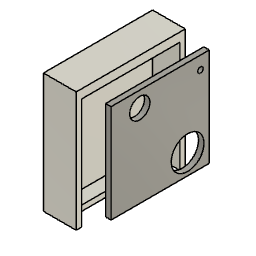
Configuration 1 (Autodesk Fusion 360 design; units mm, degrees)
Autodesk Fusion 360 part; units mm, degrees
note: some values were not read from the file. Set by a fixed rule: which sketch regions a step uses.
sketch "Sketch1" plane through (0, 0, 0) normal (1, 0, 0) x (0, 1, 0)
  line L0 (0, 0) -> (40, 0)
  line L1 (0, 0) -> (0, 43.9262)
  line L2 (0, 43.9262) -> (40, 43.9262)
  line L3 (40, 43.9262) -> (40, 0)
  dimension "d1" = 40
  constraint coincident L0.start L1.start
  constraint horizontal L0
  constraint perpendicular L0 L1
  constraint perpendicular L1 L2
  constraint perpendicular L0 L3
  measures "d1" distance of L0.start L0.end
extrude "Extrude1" add sketch "Sketch1" along normal blind 2 makes body 1
sketch "Sketch2" plane through (2, 0, 0) normal (1, 0, 0) x (0, 1, 0)
  line L0 (0, 0) -> (40, 0)
  line L1 (40, 0) -> (40, 43.9262)
  line L2 (40, 43.9262) -> (0, 43.9262)
  line L3 (0, 43.9262) -> (0, 0)
  line L4 (0, 43.9262) -> (40, 43.9262)
  line L5 (40, 0) -> (38, 0)
  line L6 (38, 40.6923) -> (2, 40.6923)
  line L7 (2, 40.6923) -> (2, 0)
  line L8 (0, 0) -> (2, 0)
  line L9 (38, 40.6923) -> (38, 0)
  constraint coincident L2.end L3.start
  constraint coincident L1.end L2.start
  constraint coincident L0.end L1.start
  constraint coincident L0 L5.end
  constraint perpendicular L1 L5
  constraint perpendicular L1 L6
  constraint coincident L0 L7.end
  constraint perpendicular L0 L7
  constraint coincident L0.start L3.end
  constraint perpendicular L5 L9
extrude "Extrude2" add sketch "Sketch2" along normal blind 10 contours L0 L1 L2 L3 L4 L5 L6 L7 L8 L9 bodies 1
sketch "Sketch3" plane through (2, 0, 0) normal (1, 0, 0) x (0, 1, 0)
  line L0 (38, 0) -> (38, 40.6923)
  line L1 (38, 40.6923) -> (2, 40.6923)
  line L2 (2, 40.6923) -> (2, 0)
  line L3 (2, 0) -> (38, 0)
  line L4 (2, 0) -> (38, 0)
  line L5 (38, 2) -> (2, 2)
  line L6 (2, 0) -> (2, 2)
  line L7 (38, 0) -> (38, 2)
  constraint coincident L2.end L3.start
  constraint coincident L0.start L3.end
  constraint coincident L2 L5.end
  constraint perpendicular L2 L5
  constraint perpendicular L5 L7
extrude "Extrude3" add sketch "Sketch3" along normal blind 5 contours L0 L2 L3 L4 L5 L6 L7 bodies 1
sketch "Sketch4" plane through (2, 0, 0) normal (1, 0, 0) x (0, 1, 0)
  line L0 (2, 2) -> (38, 2)
  line L1 (38, 2) -> (38, 40.6923)
  line L2 (38, 40.6923) -> (2, 40.6923)
  line L3 (2, 40.6923) -> (2, 2)
  line L4 (50, 0) -> (86, 0)
  line L5 (86, 0) -> (86, 36)
  line L6 (86, 36) -> (50, 36)
  line L7 (50, 36) -> (50, 0)
  dimension "d8" = 36
  dimension "d9" = 36
  constraint perpendicular L1 L4
  constraint perpendicular L4 L5
  constraint perpendicular L5 L6
  constraint perpendicular L4 L7
  measures "d8" distance of L4.start L4.end
  measures "d9" distance of L4.end L5.end
extrude "Extrude4" add sketch "Sketch4" along normal blind 2 separate body contours L4 L5 L6 L7 makes body 2
sketch "Sketch5" plane through (4, 0, 0) normal (1, 0, 0) x (0, 1, 0)
  line L0 (50, 36) -> (50, 0)
  line L1 (50, 0) -> (86, 0)
  line L2 (86, 0) -> (86, 36)
  line L3 (86, 36) -> (50, 36)
  circle A0 centre (78.0575, 7.3809) radius 6
  circle A1 centre (82.7779, 31.2818) radius 1
  dimension "d12" = 12
  dimension "d13" = 2
  measures "d12" diameter of A0
  measures "d13" diameter of A1
extrude "Extrude5" cut sketch "Sketch5" against normal blind 2 contours A0 | A1 bodies 2
move_body "Move1" bodies 2 to x (1, 0, 0) y (0, 1, 0) z (0, 0, 1) at (15, -48, 2)
move_body "Move2" bodies 2 to x (1, 0, 0) y (0, 1, 0) z (0, 0, 1) at (-6, 0, 0)
sketch "Sketch6" plane through (13, 0, 0) normal (1, 0, 0) x (0, 1, 0)
  circle A0 centre (30.0575, 9.3809) radius 6
  circle A1 centre (34.7779, 33.2818) radius 1
  line L0 (2, 38) -> (2, 2)
  line L1 (2, 2) -> (38, 2)
  line L2 (38, 2) -> (38, 38)
  line L3 (38, 38) -> (2, 38)
move_body "Move3" bodies 2 to x (1, 0, 0) y (0, 1, 0) z (0, 0, 1) at (18, 0, 0)
sketch "Sketch7" plane through (31, 0, 0) normal (1, 0, 0) x (0, 1, 0)
  circle A0 centre (30.0575, 9.3809) radius 6
  circle A1 centre (34.7779, 33.2818) radius 1
  line L0 (2, 38) -> (2, 2)
  line L1 (2, 2) -> (38, 2)
  line L2 (38, 2) -> (38, 38)
  line L3 (38, 38) -> (2, 38)
sketch "Sketch8" plane through (31, 0, 0) normal (1, 0, 0) x (0, 1, 0)
  circle A0 centre (30.0575, 9.3809) radius 6
  circle A1 centre (34.7779, 33.2818) radius 1
  line L0 (2, 38) -> (2, 2)
  line L1 (2, 2) -> (38, 2)
  line L2 (38, 2) -> (38, 38)
  line L3 (38, 38) -> (2, 38)
  circle A2 centre (12.5487, 31.9704) radius 3.725
  dimension "d18" = 7.45
  measures "d18" diameter of A2
hole "Hole1" at (31, 12.5354, 32.2776) direction (-1, 0, 0) diameter 7.45 end through all bodies 2
move_body "Move4" bodies 2 to x (1, 0, 0) y (0, 1, 0) z (0, 0, 1) at (-1.5428, 1.8094, 0.4773)
move_body "Move5" bodies 2 to x (1, 0, 0) y (0, 1, 0) z (0, 0, 1) at (0, 10, 0)
move_body "Move6" bodies 2 to x (1, 0, 0) y (0, 1, 0) z (0, 0, 1) at (-15, 0, 0)
move_body "Move7" bodies 2 to x (1, 0, 0) y (0, 1, 0) z (0, 0, 1) at (0, -12, 0)
move_body "Move8" bodies 2 to x (1, 0, 0) y (0, 1, 0) z (0, 0, 1) at (10, 0, 0)
move_body "Move9" bodies 2 to x (1, 0, 0) y (0, 1, 0) z (0, 0, 1) at (0, 15, 5)
move_body "Move10" bodies 2 to x (1, 0, 0) y (0, 1, 0) z (0, 0, 1) at (0.5173, -18.9965, -0.6609)
move_body "Move11" bodies 2 to x (1, 0, 0) y (0, 1, 0) z (0, 0, 1) at (-13, 0, 0)
move_body "Move12" bodies 2 to x (1, 0, 0) y (0, 1, 0) z (0, 0, 1) at (0, 4, 0)
move_body "Move13" bodies 2 to x (1, 0, 0) y (0, 1, 0) z (0, 0, 1) at (10, 0, 0)
move_body "Move14" bodies 2 to x (1, 0, 0) y (0, 1, 0) z (0, 0, 1) at (0, 1, 0)
named bodies: "main frame", "Cover"
